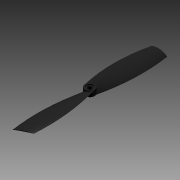
# Autodesk Inventor part: prop
Saved by Autodesk Inventor 2012 (Build 160160000, 160)
## iProperties
Created: 2014-07-09
Part Number: prop
Material: Default
Document SubType Name: Modeling
Designer: Anon
Density: 1 g/cm^3
Author: Anon
Autodesk Inventor part; units mm, degrees
ref_plane "YZ Plane" through (0, 0, 0) normal (1, 0, 0) x (0, 1, 0)
sketch "Sketch1" plane through (0, 0, 0) normal (0, 0, 1) x (1, 0, 0)
  circle A0 centre (0, 0) radius 7
  dimension "d0" = 14
  constraints: 1 centre point, 1 coincident
  measures "d0" diameter of A0
extrude "Extrusion1" add sketch "Sketch1" along normal blind 8
sketch "Sketch2" plane through (0, 0, 8) normal (0, 0, 1) x (1, 0, 0)
  circle A0 centre (0, 0) radius 7 projected
  circle A1 centre (0, 0) radius 3
  dimension "d3" = 6
  constraints: 1 centre point, 1 coincident
  measures "d3" diameter of A1
sketch "Sketch5" plane through (0, 0, 0) normal (0, 1, 0) x (-1, 0, 0)
  arc A0 (6.9886, 7.9945) -> (-5.7555, 0) centre (9.6228, -10.3597) ccw
  arc A1 (-5.7555, 0) -> (6.9886, 7.9945) centre (-13.9623, 27.2376) ccw
  point P0 (0, 0)
  constraints: 4 point on circle, 2 centre point
ref_plane "Work Plane1" through (0, 102, 0) normal (0, 1, 0) x (-1, 0, 0)
sketch "Sketch7" plane through (0, 102, 0) normal (0, 1, 0) x (-1, 0, 0)
  arc A0 (12, 2.5195) -> (-10, 0) centre (3.9145, -24.1892) ccw
  arc A1 (12, 2.5195) -> (-10, 0) centre (6.0497, -42.8334) ccw
  point P0 (0, 0)
  dimension "d32" = 12
  dimension "d33" = 10
  dimension "d34" = 0
  constraints: 4 point on circle, 2 centre point
  measures "d32" horizontal distance of A0.start point (0, 0)
  measures "d33" distance of A0.end point (0, 0)
  measures "d34" vertical distance of point (0, 0) A0.end
ref_plane "Work Plane2" through (0, 50, 0) normal (0, 1, 0) x (-1, 0, 0)
sketch "Sketch8" plane through (0, 50, 0) normal (0, 1, 0) x (-1, 0, 0)
  arc A0 (14.8793, 5.5568) -> (-12.8755, 0) centre (10.0783, -42.5555) ccw
  arc A1 (14.8793, 5.5568) -> (-12.8755, 0) centre (26.1398, -122.7786) ccw
  point P0 (0, 0)
  constraints: 4 point on circle, 2 centre point
loft "Loft1" add profiles "Sketch5", "Sketch8", "Sketch7"
pattern_circular "Circular Pattern1" count 2 over 360 about axis through (0, 0, -10) along (0, 0, 1) of "Loft1"
sketch "Sketch10" plane through (0, 0, 8) normal (0, 0, 1) x (1, 0, 0)
  circle A0 centre (0, 0) radius 7 projected
  circle A1 centre (0, 0) radius 102
  circle A2 centre (0, 0) radius 119.0756
  dimension "d25" = 204
  constraints: 2 centre point, 2 coincident
  measures "d25" diameter of A1
extrude "Extrusion4" cut sketch "Sketch10" against normal through all contours A2
sketch "Sketch11" plane through (0, 0, 8) normal (0, 0, 1) x (1, 0, 0)
  arc A0 (-9.2755, -101.2344) -> (21.1659, -88.2344) centre (-16.6676, -41.7833) ccw
  line L0 (21.1659, -88.2344) -> (21.1659, -103.2344)
  line L1 (21.1659, -103.2344) -> (-9.2755, -103.2344)
  line L2 (-9.2755, -101.2344) -> (-9.2755, -103.2344)
  dimension "d28" = 15
  dimension "d29" = 2
  constraints: 6 end point, 2 perpendicular, 2 point on circle, 1 centre point, 1 vertical
  measures "d28" distance of L0.start L0.end
  measures "d29" distance of L2.start L1.end
extrude "Extrusion5" cut sketch "Sketch11" against normal through all
sketch "Sketch3" plane through (0, 0, 8) normal (0, 0, 1) x (1, 0, 0)
  circle A0 centre (0, 0) radius 3 projected
  circle A1 centre (0, 0) radius 7 projected
  circle A2 centre (0, 0) radius 5
  dimension "d6" = 10
  constraints: 1 centre point, 1 coincident
  measures "d6" diameter of A2
extrude "Extrusion6" cut sketch "Sketch3" against normal through all contours A0
sketch "Sketch12" plane through (0, 0, 8) normal (0, 0, 1) x (1, 0, 0)
  circle A0 centre (0, 0) radius 3 projected
  circle A1 centre (0, 0) radius 7 projected
  circle A2 centre (0, 0) radius 5
  dimension "d37" = 10
  constraints: 1 centre point, 1 coincident
  measures "d37" diameter of A2
extrude "Extrusion7" cut sketch "Sketch12" against normal blind 1.3 contours A2
body "Solid1"
